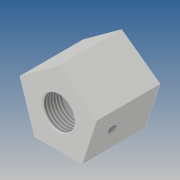
# Autodesk Inventor part: ammo_blocker
Saved by Autodesk Inventor 2019 (Build 230136000, 136)
## iProperties
Created: 2019-03-08
Part Number: ammo_blocker
Material: Générique
Document SubType Name: Modeling
Designer: Theo
Density: 1 g/cm^3
Appearance: Par défaut
Author: Theo
Autodesk Inventor part; units mm, degrees
ref_plane "YZ Plane" through (0, 0, 0) normal (1, 0, 0) x (0, 1, 0)
ref_plane "XZ Plane" through (0, 0, 0) normal (0, 1, 0) x (-1, 0, 0)
ref_plane "XY Plane" through (0, 0, 0) normal (0, 0, 1) x (1, 0, 0)
sketch "Esquisse2" plane through (0, 0, 0) normal (1, 0, 0) x (0, 1, 0)
  line L0 (6.25, -10) -> (6.25, -11)
  line L1 (6.25, -11) -> (9.5, -21)
  line L2 (9.5, -21) -> (9.5, -31)
  line L3 (0, -252.0623) -> (0, 0)
  line L4 (9.5, -31) -> (12.5, -31)
  line L5 (12.5, -31) -> (12.5, 0)
  line L6 (6.25, -10) -> (7.75, -10)
  line L7 (12.5, 0) -> (7.75, 0)
  line L8 (7.75, 0) -> (7.75, -10)
  dimension "d1" = 10
  dimension "d4" = 12.5
  dimension "d6" = 3
  dimension "d8" = 1.5
  dimension "d11" = 19
  dimension "d12" = 20
  dimension "d15" = 25
  dimension "d16" = 1
  dimension "d17" = 10
  dimension "d22" = 15.5
  constraints: 18 end point, 5 vertical, 3 horizontal, 1 horizontal alignment
  measures "d1" vertical distance of L0.end L1.end
  measures "d4" diameter of L0 L3
  measures "d6" distance of L2.end L4.end
  measures "d8" distance of L0.start L6.end
  measures "d11" diameter of L2 L3
  measures "d12" distance from line of L4 L0.end
  measures "d15" diameter of L5.end L3
  measures "d16" distance of L0.start L0.end
  measures "d17" distance of L7.end L6.end
  measures "d22" diameter of L7.end L3
revolve "Révolution1" add sketch "Esquisse2" angle 360 about axis through (0, 0, -252.0623) along (0, 0, 1)
thread "Filetage3" size "M16x1.5" class "6H" standard "ISO Metric profile" full length
chamfer "Chanfrein1" distance 0.5 angle 45 1 edges at (0, -7.75, 0)
sketch "Esquisse7" plane through (0, 0, -31) normal (0, 0, -1) x (-1, 0, 0)
  line L0 (-11.6247, -16) -> (-18.8091, 6.1115)
  line L1 (-18.8091, 6.1115) -> (0, 19.7771)
  line L2 (0, 19.7771) -> (18.8091, 6.1115)
  line L3 (18.8091, 6.1115) -> (11.6247, -16)
  line L4 (11.6247, -16) -> (-11.6247, -16)
  circle A0 centre (0, 0) radius 12.5 projected
  circle A1 centre (0, 0) radius 9.5 projected
  dimension "d44" = 16
  constraints: 10 end point, 1 coincident, 1 horizontal, 11 other
  measures "d44" distance from line of point (0, 0) L4
extrude "Extrusion5" add sketch "Esquisse7" against normal up to surface (31 mm away) contours L0 L1 L2 L3 L4
sketch "Esquisse8" plane through (11.6247, -16, 0) normal (0.9511, -0.309, 0) x (0, 0, -1)
  line L0 (21, 2.1247) -> (21, 21.1247) projected
  line L1 (11, 5.3747) -> (11, 17.8747) projected
  line L2 (10, 5.3747) -> (10, 17.8747) projected
  point P0 (0, 11.6247)
  point P1 (11, 11.6247)
  point P2 (11, 11.6247)
  constraints: 2 coincident, 1 midpoint
hole "Perçage2" at (15.2169, -4.9443, -11) direction (-0.9511, 0.309, 0) diameter 4.134 depth 7 tip angle 118 thread size "M5x0.8" class "6H" standard "ISO Metric profile"
mirror "Symétrie1" about plane through (0, 0, 0) normal (1, 0, 0) of "Perçage2"
chamfer "Chanfrein2" distance 4 angle 45 1 edges at (0, -9.5, -31)
